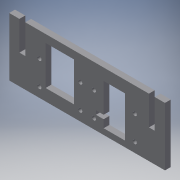
# Autodesk Inventor part: Camera bracket
Saved by Autodesk Inventor 2018 (Build 220112000, 112)
## iProperties
Created: 2018-05-02
Part Number: Camera bracket
Material: Generic
Document SubType Name: Modeling
Designer: Ajith Thomas
Density: 1 g/cm^3
Appearance: Default
Author: Ajith Thomas
Autodesk Inventor part; units mm, degrees
ref_plane "YZ Plane" through (0, 0, 0) normal (1, 0, 0) x (0, 1, 0)
ref_plane "XZ Plane" through (0, 0, 0) normal (0, 1, 0) x (-1, 0, 0)
ref_plane "XY Plane" through (0, 0, 0) normal (0, 0, 1) x (1, 0, 0)
sketch "Sketch1" plane through (0, 0, 0) normal (0, 0, 1) x (1, 0, 0)
  line L0 (-12.5, 9.5) -> (-12.5, -14.5) construction
  line L1 (-15.5, -14.5) -> (-15.5, 9.5) construction
  line L2 (-12.5, -2.5) -> (-15.5, -2.5) construction
  line L3 (26, -17.5) -> (-54, -17.5)
  line L4 (-54, -17.5) -> (-54, 12.5)
  line L5 (-54, 12.5) -> (26, 12.5)
  line L6 (26, 12.5) -> (26, -17.5)
  line L7 (26, -17.5) -> (-54, 12.5) construction
  line L8 (-54, -17.5) -> (26, 12.5) construction
  line L9 (-12.5, -14.5) -> (12.5, -14.5) construction
  line L10 (12.5, -14.5) -> (12.5, 9.5) construction
  line L11 (12.5, 9.5) -> (-12.5, 9.5) construction
  line L12 (-15.5, 9.5) -> (-40.5, 9.5) construction
  line L13 (-40.5, 9.5) -> (-40.5, -14.5) construction
  line L14 (-40.5, -14.5) -> (-15.5, -14.5) construction
  line L15 (-8.7, -9.1) -> (-8.7, -9.9) construction
  line L16 (-8.7, -9.9) -> (-7.48, -9.9) construction
  line L17 (-7.48, -9.9) -> (-7.48, -9.1) construction
  line L18 (-7.48, -9.1) -> (-8.7, -9.1) construction
  circle A0 centre (-10.5, -12.5) radius 1.05 projected
  circle A1 centre (-10.5, 0) radius 1.05 projected
  circle A2 centre (10.5, 0) radius 1.05 projected
  circle A3 centre (10.5, -12.5) radius 1.05 projected
  circle A4 centre (-17.5, -12.5) radius 1.05 projected
  circle A5 centre (-17.5, 0) radius 1.05 projected
  circle A6 centre (-38.5, -12.5) radius 1.05 projected
  circle A7 centre (-38.5, 0) radius 1.05 projected
  line L19 (5.5, -14.5) -> (-5.5, -14.5)
  line L20 (5.5, 6.5) -> (5.5, -14.5)
  line L21 (-5.5, -10.5) -> (-9.45, -10.5)
  line L22 (-5.5, -8.5) -> (-9.45, -8.5)
  line L23 (-9.45, -10.5) -> (-9.45, -8.5)
  line L24 (-5.5, -14.5) -> (-5.5, -10.5)
  line L25 (-5.5, -8.5) -> (-5.5, 6.5)
  line L26 (-35.3, -11.5) -> (-35.3, 8.5)
  line L27 (-20.7, 8.5) -> (-20.7, -11.5)
  line L28 (5.5, 6.5) -> (-5.5, 6.5)
  line L29 (-20.7, -11.5) -> (-35.3, -11.5)
  line L30 (-20.7, 8.5) -> (-35.3, 8.5)
  line L31 (20.75, 12.5) -> (17.75, 12.5)
  line L32 (17.75, 12.5) -> (17.75, -2.5)
  line L33 (17.75, -2.5) -> (20.75, -2.5)
  line L34 (20.75, -2.5) -> (20.75, 12.5)
  line L35 (-14, -17.5) -> (-14, 12.5) construction
  line L36 (-48.75, 12.5) -> (-45.75, 12.5)
  line L37 (-45.75, 12.5) -> (-45.75, -2.5)
  line L38 (-45.75, -2.5) -> (-48.75, -2.5)
  line L39 (-48.75, -2.5) -> (-48.75, 12.5)
  point P0 (0, 0)
  point P1 (-14, -2.5)
  dimension "d0" = 80
  dimension "d1" = 30
  dimension "d2" = 7
  dimension "d4" = 4
  dimension "d6" = 18
  dimension "d7" = 7
  dimension "d8" = 7
  dimension "d9" = 3.05
  dimension "d10" = 3
  dimension "d11" = 5.2
  dimension "d12" = 5.2
  dimension "d13" = 3
  dimension "d14" = 3
  dimension "d15" = 1
  dimension "d16" = 15
  dimension "d17" = 5.25
  dimension "d18" = 13.5
  dimension "d19" = 3
  constraints: 56 end point, 10 perpendicular, 7 midpoint, 7 parallel, 4 symmetric about line, 3 horizontal, 2 point on line
  measures "d0" distance of L4.end L5.end
  measures "d1" distance of L3.end L4.end
  measures "d2" distance between parallel lines of L10 L20
  measures "d4" distance between parallel lines of L9 L21
  measures "d6" distance between parallel lines of L11 L22
  measures "d7" distance between parallel lines of L0 L25
  measures "d8" distance between parallel lines of L0 L24
  measures "d9" distance between parallel lines of L0 L23
  measures "d10" distance between parallel lines of L3 L19
  measures "d11" distance between parallel lines of L1 L27
  measures "d12" distance between parallel lines of L13 L26
  measures "d13" distance between parallel lines of L11 L28
  measures "d14" distance between parallel lines of L14 L29
  measures "d15" distance between parallel lines of L12 L30
  measures "d16" distance between parallel lines of L5 L33
  measures "d17" distance between parallel lines of L6 L34
  measures "d18" distance between parallel lines of L10 L6
  measures "d19" distance between parallel lines of L32 L34
extrude "Extrusion1" add sketch "Sketch1" along normal blind 3 contours L3 L4 L5 L39 L38 L37 L32 L33 L34 L6
body "Solid1"
